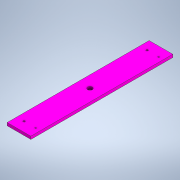
# Autodesk Inventor part: Estabilizador
Saved by Autodesk Inventor 2022 (Build 260153000, 153)
## iProperties
Created: 2022-03-01
Part Number: Estabilizador
Material: Generic
Document SubType Name: Modeling
Designer: Home
Density: 1 g/cm^3
Appearance: Default
Author: Home
Autodesk Inventor part; units mm, degrees
ref_plane "YZ Plane" through (0, 0, 0) normal (1, 0, 0) x (0, 1, 0)
ref_plane "XZ Plane" through (0, 0, 0) normal (0, 1, 0) x (-1, 0, 0)
ref_plane "XY Plane" through (0, 0, 0) normal (0, 0, 1) x (1, 0, 0)
sketch "Sketch1" plane through (0, 0, 0) normal (0, 1, 0) x (-1, 0, 0)
  circle A0 centre (0, 0) radius 5
  circle A1 centre (9.4, 130) radius 2
  circle A2 centre (9.4, -130) radius 2
  line L0 (25, 150) -> (-25, 150)
  line L1 (-25, 150) -> (-25, -150)
  line L2 (-25, -150) -> (25, -150)
  line L3 (25, -150) -> (25, 150)
  line L4 (25, 150) -> (-25, -150) construction
  line L5 (-25, 150) -> (25, -150) construction
  circle A3 centre (-15, 130) radius 1.5
  circle A4 centre (-15, -130) radius 1.5
  dimension "d0" = 10
  dimension "d3" = 4
  dimension "d4" = 4
  dimension "d6" = 50
  dimension "d7" = 300
  dimension "d9" = 9.4
  dimension "d11" = 260
  dimension "d12" = 20
  dimension "d15" = 3
  dimension "d16" = 10
  dimension "d17" = 3
  constraints: 12 end point, 5 centre point, 2 horizontal alignment, 2 midpoint, 2 parallel, 2 vertical alignment, 1 coincident, 1 horizontal, 1 perpendicular
  measures "d0" diameter of A0
  measures "d3" diameter of A1
  measures "d4" diameter of A2
  measures "d6" distance of L2.end L1.end
  measures "d7" distance of L1.end L0.end
  measures "d9" horizontal distance of A1.centre point (0, 0)
  measures "d11" distance of A1.centre A2.centre
  measures "d12" distance from line of L0 A1.centre
  measures "d15" diameter of A3
  measures "d16" distance from line of A3.centre L1
  measures "d17" diameter of A4
extrude "Extrusion2" add sketch "Sketch1" along normal blind 6
body "Solid2"
